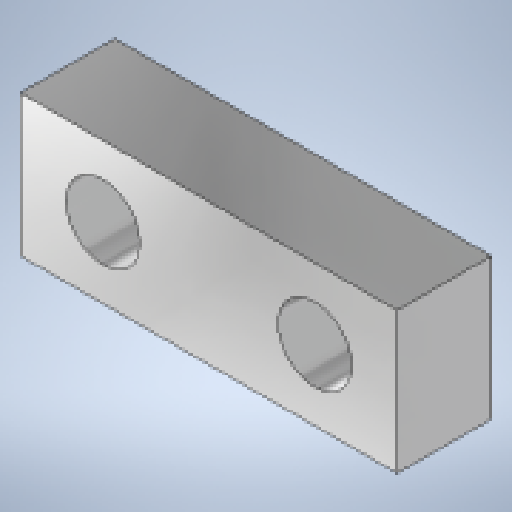
# Autodesk Inventor part: Arms
Saved by Autodesk Inventor 2023.2 (Build 272271000, 271)
## iProperties
Created: 2024-02-19
Part Number: Arms
Material: Aluminum 6061
Document SubType Name: Modeling
Designer: Nathan Cai
Density: 2.7 g/cm^3
Appearance: Aluminum - Flat
Author: Nathan Cai
Autodesk Inventor part; units mm, degrees
ref_plane "YZ Plane" through (0, 0, 0) normal (1, 0, 0) x (0, 1, 0)
ref_plane "XZ Plane" through (0, 0, 0) normal (0, 1, 0) x (-1, 0, 0)
ref_plane "XY Plane" through (0, 0, 0) normal (0, 0, 1) x (1, 0, 0)
sketch "Sketch1" plane through (0, 0, 0) normal (0, 0, 1) x (1, 0, 0)
  line L0 (12.7, -4.7625) -> (-12.7, -4.7625)
  line L1 (-12.7, -4.7625) -> (-12.7, 4.7625)
  line L2 (-12.7, 4.7625) -> (12.7, 4.7625)
  line L3 (12.7, 4.7625) -> (12.7, -4.7625)
  line L4 (12.7, -4.7625) -> (-12.7, 4.7625) construction
  line L5 (-12.7, -4.7625) -> (12.7, 4.7625) construction
  line L6 (-12.7, 0) -> (12.7, 0) construction
  circle A0 centre (-7.1437, 0) radius 2.4892
  line L7 (0, -4.7625) -> (0, 4.7625) construction
  circle A1 centre (7.1437, 0) radius 2.4892
  point P0 (0, 0)
  point P1 (0, 0)
  dimension "d0" = 25.4
  dimension "d1" = 9.525
  dimension "d2" = 4.9784
  dimension "d3" = 7.1437
  constraints: 16 end point, 7 midpoint, 2 centre point, 2 parallel, 1 horizontal, 1 perpendicular, 1 point on line, 1 symmetric about line, 1 other
  measures "d0" distance of L1.end L2.end
  measures "d1" distance of L0.end L1.end
  measures "d2" diameter of A0
  measures "d3" distance of point (0, 0) A0.centre
extrude "Extrusion1" add sketch "Sketch1" along normal blind 6.35
body "Solid1"
